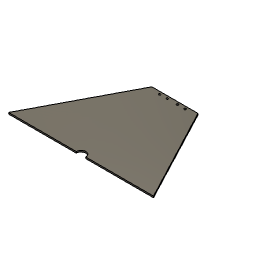
Front (Autodesk Fusion 360 design; units mm, degrees)
Autodesk Fusion 360 part; units mm, degrees
note: some values were not read from the file. Set by a fixed rule: which sketch regions a step uses.
sketch "Sketch1" plane through (0, 0, 0) normal (0, 1, 0) x (1, 0, 0)
  line L0 (155.2575, 192.4304) -> (109.5375, 192.4304)
  line L1 (155.2575, 192.4304) -> (200.9775, 192.4304)
  circle A0 centre (145.0975, 187.3504) radius 1.905
  circle A1 centre (129.8575, 187.3504) radius 1.905
  circle A2 centre (165.4175, 187.3504) radius 1.905
  circle A3 centre (180.6575, 187.3504) radius 1.905
  arc A4 (164.7825, 6) -> (145.7325, 6) centre (155.2575, 6) ccw
  line L2 (299.0996, 6) -> (164.7825, 6)
  line L3 (145.7325, 6) -> (11.4154, 6)
  line L4 (11.4154, 6) -> (109.5375, 192.4304)
  line L5 (299.0996, 6) -> (200.9775, 192.4304)
  dimension "d3" = 45.72
  dimension "d4" = 45.72
  dimension "d22" = 19.05
  constraint horizontal L2
  constraint coincident A4.end L2
  constraint collinear L2 L3
  constraint coincident A4.centre L2
  measures "d3" distance of L0.start L0.end
  measures "d4" distance of L0.start L1.end
  measures "d22" diameter of A4
extrude "Extrude3" add sketch "Sketch1" along normal blind 2.794
equation "d3 = ( 3.6 / 2 ) * 1 in"
equation "d4 = ( 3.6 / 2 ) * 1 in"
